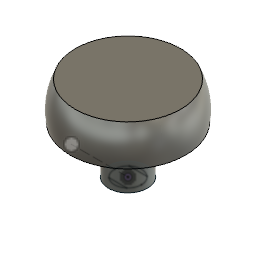
OpenMicroJoystickCap (Autodesk Fusion 360 design; units mm, degrees)
Autodesk Fusion 360 part; units mm, degrees
note: some values were not read from the file. Chosen so that the rebuilt part matches the saved one: which sketch regions a step uses.
sketch "Sketch1" plane through (0, 0, 0) normal (0, 0, 1) x (1, 0, 0)
  circle A0 centre (0, 9) radius 9
  circle A1 centre (0, -15) radius 24
  line L0 (-3, 0) -> (3, 0)
  line L1 (3, 0) -> (3, 9)
  line L2 (3, 9) -> (-3, 9)
  line L3 (-3, 9) -> (-3, 0)
  line L4 (0, 0) -> (0, 41) construction
  line L5 (0, 0) -> (0, 8)
  line L6 (-8.0623, 13) -> (8.0623, 13)
  line L7 (0, 13) -> (0, 0)
  dimension "d1" = 18
  dimension "d2" = 6
  dimension "d4" = 48
  dimension "d5" = 9
  dimension "d17" = 13
  constraint horizontal L0
  constraint vertical L1
  constraint horizontal L2
  constraint vertical L3
  constraint coincident L4.start L5.start
  constraint perpendicular L0 L4
  constraint symmetric L1 L3 L4
  constraint coincident A0.centre L2
  constraint coincident A0.centre A1
  constraint coincident L4.start L0
  constraint coincident L4 L5.end
  constraint coincident A0.centre L4
  constraint coincident A1.centre L4
  constraint coincident A0 L6.start
  constraint coincident A0 L6.end
  constraint horizontal L6
  constraint midpoint L6 L7.start
  measures "d1" diameter of A0
  measures "d2" distance of L1 L3
  measures "d4" diameter of A1
  measures "d5" distance of L0.end L1.end
  measures "d17" distance of L4.start L6
revolve "Revolve1" add sketch "Sketch1" angle 360 about axis through (0, 0, 0) along (0, 1, 0) contours A0 A1 L1 L2 L6 L7 | A0 L0 L1 | A0 A1 L1 L5 L7 | A1 L1 L2 | A1 L2 L3
sketch "Sketch2" plane through (0, 0, 0) normal (0, -1, 0) x (1, 0, 0)
  circle A0 centre (0, 0) radius 3
  circle A1 centre (0, 0) radius 2.05
  line L0 (-1.3416, 1.55) -> (1.3416, 1.55)
  line L1 (-1.3416, -1.55) -> (1.3416, -1.55)
  line L2 (0, 0) -> (-8.6502, 0) construction
  dimension "d8" = 4.1
  dimension "d9" = 3.1
  constraint coincident A0.centre A1.centre
  constraint coincident A1 L0.start
  constraint coincident A1 L0.end
  constraint horizontal L0
  constraint coincident A1 L1.start
  constraint coincident A1 L1.end
  constraint parallel L0 L1
  constraint parallel L1 L2
  constraint symmetric L0 L1 L2
  measures "d8" diameter of A1
  measures "d9" distance of L0 L1
extrude "Extrude1" [suppressed]
sketch "Sketch3" plane through (0, 5, 0) normal (0, -1, 0) x (1, 0, 0)
  arc A0 (-1.3229, 1.5) -> (-1.3229, -1.5) centre (0, 0) ccw
  line L0 (-1.3229, -1.5) -> (1.3229, -1.5)
  arc A1 (1.3229, -1.5) -> (1.3229, 1.5) centre (0, 0) ccw
  line L1 (1.3229, 1.5) -> (-1.3229, 1.5)
  circle A2 centre (0, 0) radius 0.55
  dimension "d12" = 1.1
  constraint coincident A0.centre A1.centre
  measures "d12" diameter of A2
extrude "Extrude2" [suppressed]
fillet "Fillet1" [suppressed]
fillet "Fillet2" [suppressed]
